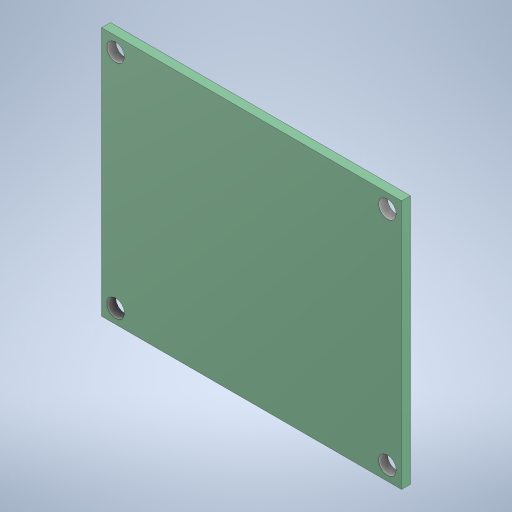
# Autodesk Inventor part: Board_Main
Saved by Autodesk Inventor 2023 (Build 270158000, 158)
## iProperties
Created: 2023-03-15
Part Number: Board_Main
Material: Generic
Document SubType Name: Modeling
Designer: karpova
Density: 1 g/cm^3
Appearance: Default
Author: karpova
Autodesk Inventor part; units mm, degrees
ref_plane "YZ Plane" through (0, 0, 0) normal (1, 0, 0) x (0, 1, 0)
ref_plane "XZ Plane" through (0, 0, 0) normal (0, 1, 0) x (-1, 0, 0)
ref_plane "XY Plane" through (0, 0, 0) normal (0, 0, 1) x (1, 0, 0)
sketch "Sketch1" plane through (0, 0, 0) normal (0, 0, 1) x (1, 0, 0)
  line L0 (0, 0) -> (54, 0)
  line L1 (54, 0) -> (54, 45)
  line L2 (54, 45) -> (0, 45)
  line L3 (0, 45) -> (0, 0)
  dimension "d0" = 54
  dimension "d1" = 45
  constraints: 8 end point, 2 parallel, 1 horizontal, 1 perpendicular
  measures "d0" distance of L1.end L2.end
  measures "d1" distance of L2.end L0.start
extrude "Extrusion1" add sketch "Sketch1" along normal blind 1.5875
sketch "Sketch2" plane through (0, 0, 1.5875) normal (0, 0, 1) x (1, 0, 0)
  line L0 (2.5398, 42.4644) -> (2.5398, 2.5356) construction
  line L1 (2.5398, 2.5356) -> (51.4602, 2.5356) construction
  line L2 (51.4602, 2.5356) -> (51.4602, 42.4644) construction
  line L3 (51.4602, 42.4644) -> (2.5398, 42.4644) construction
  line L4 (27, 2.5356) -> (27, 42.4644) construction
  line L5 (2.5398, 22.5) -> (51.4602, 22.5) construction
  line L6 (54, 0) -> (54, 45) construction
  line L7 (54, 45) -> (0, 45) construction
  line L8 (0, 45) -> (0, 0) construction
  line L9 (0, 0) -> (54, 0) construction
  line L10 (27, 0) -> (27, 45) construction
  line L11 (0, 22.5) -> (54, 22.5) construction
  dimension "d4" = 39.9288
  dimension "d5" = 48.9204
  constraints: 16 end point, 8 midpoint, 3 perpendicular, 2 collinear, 1 horizontal
  measures "d4" distance of L0.end L0.start
  measures "d5" distance of L1.end L0.end
hole "Hole1" at (2.5398, 2.5356, 1.5875) at (2.5398, 42.4644, 1.5875) at (51.4602, 42.4644, 1.5875) at (51.4602, 2.5356, 1.5875) direction (0, 0, -1) diameter 3.175 end through all
body "Solid1"
